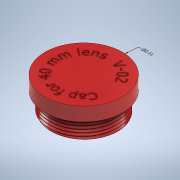
# Autodesk Inventor part: CapForSvBonyPlosse-40mm-V02
Saved by Autodesk Inventor 2021.1 (Build 251245010, 245A)
## iProperties
Created: 2020-10-08
Part Number: CapForSvBonyPlosse-40mm-V02
Material: PC/ABS Plastic
Document SubType Name: Modeling
Designer: robst
Density: 0.357273 g/cm^3
Appearance: Red
Author: robst
Autodesk Inventor part; units mm, degrees
ref_plane "YZ Plane" through (0, 0, 0) normal (1, 0, 0) x (0, 1, 0)
ref_plane "XZ Plane" through (0, 0, 0) normal (0, 1, 0) x (-1, 0, 0)
ref_plane "XY Plane" through (0, 0, 0) normal (0, 0, 1) x (1, 0, 0)
sketch "Sketch7" plane through (0, 0, 0) normal (0, 0, 1) x (1, 0, 0)
  line L0 (0, 0) -> (23.5712, 0)
  line L1 (23.5712, 0) -> (23.5712, 12.7)
  line L2 (23.5712, 12.7) -> (26.7462, 12.7)
  line L3 (26.7462, 12.7) -> (26.7462, 22.225)
  line L4 (26.7462, 22.225) -> (0, 22.225)
  line L5 (23.5712, 0) -> (20.3962, 0)
  line L6 (20.3962, 0) -> (20.3962, 19.05)
  line L7 (20.3962, 19.05) -> (0, 19.05)
  line L8 (0, 22.225) -> (0, 19.05)
  line L9 (0, -4.445) -> (0, 26.67) projected
  dimension "d71" = 9.525
  dimension "d72" = 12.7
  dimension "d73" = 23.5712
  dimension "d77" = 3.175
  dimension "d78" = 3.175
  dimension "d117" = 20.3962
  constraints: 18 end point, 5 perpendicular, 2 vertical, 1 horizontal, 1 point on line
  measures "d71" distance between parallel lines of L4 L2
  measures "d72" distance from line of L2 L0.start
  measures "d73" distance of L0.start L0.end
  measures "d77" distance of L2.end L1.end
  measures "d78" distance between parallel lines of L1 L6
  measures "d117" distance between parallel lines of L6 L9
revolve "Revolution3" add sketch "Sketch7" angle 360 about axis through (0, -10, 0) along (0, 1, 0) contours L6 L7 L8 L4 L3 L2 L1 L0
sketch "Sketch10" plane through (0, 0, 0) normal (0, 0, 1) x (1, 0, 0)
  line L0 (23.5712, 12.7) -> (23.5712, 0) projected
  line L1 (23.5712, -2.1167) -> (23.5712, -4.0025)
  line L2 (23.5712, -4.0025) -> (22.3266, -3.284)
  line L3 (22.3266, -2.8352) -> (23.5712, -2.1167)
  line L4 (-23.5712, 0) -> (23.5712, 0) projected
  arc A0 (22.3266, -2.8352) -> (22.3266, -3.284) centre (22.4561, -3.0596) ccw
  line L5 (0, -7.3431) -> (0, 16.0405) projected
  point P0 (0, 0)
  dimension "d100" = 60
  dimension "d101" = 2.1167
  dimension "d102" = 0.2591
  dimension "d103" = 22.1971
  constraints: 6 end point, 2 point on circle, 2 tangent, 1 centre point, 1 collinear, 1 equal length, 1 vertical
  measures "d100" angle of L3 L2
  measures "d101" distance from line of L1.start L4
  measures "d102" radius of A0
  measures "d103" distance edge to line of A0 L5
coil "Coil6" sketch "Sketch10" operation cut axis through (0, -10, 0) along (0, 1, 0) pitch 2.1167 turns 8 hand right
sketch "Sketch11" plane through (0, 22.225, 0) normal (0, 1, 0) x (1, 0, 0)
  circle A0 centre (0, 0) radius 19.05 construction
  spline S0 degree 2 poles (13.5686, -8.6606) (13.8543, -8.1839) (14.6595, -7.5704) (15.1574, -7.4694) knots 0 0 0 1 2 2 2
  spline S1 degree 2 poles (15.1574, -7.4694) (15.6514, -7.3659) (16.7976, -7.6157) (17.4173, -7.9871) knots 0 0 0 1 2 2 2
  spline S2 degree 2 poles (17.4173, -7.9871) (18.033, -8.3562) (18.7585, -9.2177) (18.9175, -9.718) knots 0 0 0 1 2 2 2
  spline S3 degree 2 poles (18.9175, -9.718) (19.071, -10.2096) (18.9356, -11.2192) (18.6379, -11.7157) knots 0 0 0 1 2 2 2
  spline S4 degree 2 poles (18.6379, -11.7157) (18.4903, -11.962) (18.1592, -12.3521) (17.9941, -12.5015) knots 0 0 0 1 2 2 2
  spline S5 degree 2 poles (17.9941, -12.5015) (17.8472, -12.6294) (17.5026, -12.871) (17.3175, -12.9815) knots 0 0 0 1 2 2 2
  line L0 (17.3175, -12.9815) -> (16.5311, -12.51)
  line L1 (16.5311, -12.51) -> (16.562, -12.4583)
  spline S6 degree 2 poles (16.562, -12.4583) (16.6938, -12.4186) (17.0782, -12.2818) (17.3021, -12.1515) knots 0 0 0 1 2 2 2
  spline S7 degree 2 poles (17.3021, -12.1515) (17.5173, -12.0267) (17.9127, -11.6644) (18.0842, -11.3784) knots 0 0 0 1 2 2 2
  spline S8 degree 2 poles (18.0842, -11.3784) (18.2723, -11.0646) (18.3499, -10.3497) (18.2298, -9.9915) knots 0 0 0 1 2 2 2
  spline S9 degree 2 poles (18.2298, -9.9915) (18.1034, -9.635) (17.4828, -8.9498) (17.0101, -8.6664) knots 0 0 0 1 2 2 2
  spline S10 degree 2 poles (17.0101, -8.6664) (16.5056, -8.364) (15.6335, -8.1705) (15.257, -8.231) knots 0 0 0 1 2 2 2
  spline S11 degree 2 poles (15.257, -8.231) (14.8909, -8.2923) (14.3136, -8.6968) (14.1279, -9.0066) knots 0 0 0 1 2 2 2
  spline S12 degree 2 poles (14.1279, -9.0066) (13.9588, -9.2887) (13.8097, -9.8526) (13.8011, -10.1012) knots 0 0 0 1 2 2 2
  spline S13 degree 2 poles (13.8011, -10.1012) (13.7972, -10.3419) (13.8521, -10.7366) (13.8824, -10.8574) knots 0 0 0 1 2 2 2
  line L2 (13.8824, -10.8574) -> (13.8538, -10.905)
  line L3 (13.8538, -10.905) -> (13.0752, -10.4383)
  spline S14 degree 2 poles (13.0752, -10.4383) (13.0974, -10.2302) (13.1298, -9.8608) (13.1877, -9.6202) knots 0 0 0 1 2 2 2
  spline S15 degree 2 poles (13.1877, -9.6202) (13.2448, -9.3628) (13.3924, -8.9545) (13.5686, -8.6606) knots 0 0 0 1 2 2 2
  spline S16 degree 2 poles (10.8434, -12.6588) (10.8626, -12.5511) (10.9182, -12.1791) (10.9711, -12.0331) knots 0 0 0 1 2 2 2
  spline S17 degree 2 poles (10.9711, -12.0331) (11.0387, -11.8285) (11.224, -11.5057) (11.4592, -11.2825) knots 0 0 0 1 2 2 2
  spline S18 degree 2 poles (11.4592, -11.2825) (11.6506, -11.1008) (12.1337, -10.9169) (12.3891, -10.9235) knots 0 0 0 1 2 2 2
  spline S19 degree 2 poles (12.3891, -10.9235) (12.6345, -10.9332) (13.1427, -11.1659) (13.3404, -11.3742) knots 0 0 0 1 2 2 2
  spline S20 degree 2 poles (13.3404, -11.3742) (13.6465, -11.6967) (13.808, -12.4118) (13.6368, -12.8233) knots 0 0 0 1 2 2 2
  spline S21 degree 2 poles (13.6368, -12.8233) (13.4895, -13.193) (12.8635, -13.9596) (12.4726, -14.3753) knots 0 0 0 1 2 2 2
  line L4 (12.4726, -14.3753) -> (12.5683, -14.476)
  spline S22 degree 2 poles (12.5683, -14.476) (12.7405, -14.6574) (13.0649, -14.7773) (13.2263, -14.7454) knots 0 0 0 1 2 2 2
  spline S23 degree 2 poles (13.2263, -14.7454) (13.3876, -14.7136) (13.7148, -14.4797) (13.8693, -14.3331) knots 0 0 0 1 2 2 2
  spline S24 degree 2 poles (13.8693, -14.3331) (14.0507, -14.1609) (14.4391, -13.5879) (14.5854, -13.251) knots 0 0 0 1 2 2 2
  line L5 (14.5854, -13.251) -> (14.6157, -13.2223)
  line L6 (14.6157, -13.2223) -> (15.1226, -13.7564)
  spline S25 degree 2 poles (15.1226, -13.7564) (15.0164, -13.9338) (14.5713, -14.5479) (14.3059, -14.7998) knots 0 0 0 1 2 2 2
  spline S26 degree 2 poles (14.3059, -14.7998) (13.9834, -15.1059) (13.4477, -15.4228) (13.1487, -15.4576) knots 0 0 0 1 2 2 2
  spline S27 degree 2 poles (13.1487, -15.4576) (12.8563, -15.4925) (12.3025, -15.2455) (12.0251, -14.9532) knots 0 0 0 1 2 2 2
  line L7 (12.0251, -14.9532) -> (10.0069, -12.8269)
  line L8 (10.0069, -12.8269) -> (10.531, -12.3296)
  line L9 (10.531, -12.3296) -> (10.8434, -12.6588)
  line L10 (11.2579, -13.0954) -> (12.0773, -13.9587)
  spline S28 degree 2 poles (12.0773, -13.9587) (12.2495, -13.7634) (12.7629, -13.1675) (12.89, -12.9447) knots 0 0 0 1 2 2 2
  spline S29 degree 2 poles (12.89, -12.9447) (13.0376, -12.6832) (13.0579, -12.1596) (12.8347, -11.9245) knots 0 0 0 1 2 2 2
  spline S30 degree 2 poles (12.8347, -11.9245) (12.5796, -11.6557) (12.019, -11.6706) (11.7302, -11.9448) knots 0 0 0 1 2 2 2
  spline S31 degree 2 poles (11.7302, -11.9448) (11.4849, -12.1775) (11.2827, -12.7718) (11.2579, -13.0954) knots 0 0 0 1 2 2 2
  spline S32 degree 2 poles (7.1265, -17.1316) (6.6121, -16.1883) (6.9032, -14.5842) (7.5904, -14.2095) knots 0 0 0 1 2 2 2
  spline S33 degree 2 poles (7.5904, -14.2095) (7.8709, -14.0565) (8.3729, -13.9516) (8.6697, -13.9638) knots 0 0 0 1 2 2 2
  line L11 (8.6697, -13.9638) -> (7.8094, -12.3862)
  line L12 (7.8094, -12.3862) -> (8.4437, -12.0403)
  line L13 (8.4437, -12.0403) -> (11.2529, -17.192)
  line L14 (11.2529, -17.192) -> (10.6186, -17.5379)
  line L15 (10.6186, -17.5379) -> (10.4036, -17.1435)
  spline S34 degree 2 poles (10.4036, -17.1435) (10.2853, -17.4876) (9.8631, -18.087) (9.5256, -18.2711) knots 0 0 0 1 2 2 2
  spline S35 degree 2 poles (9.5256, -18.2711) (8.8791, -18.6236) (7.5966, -17.9936) (7.1265, -17.1316) knots 0 0 0 1 2 2 2
  spline S36 degree 2 poles (7.7413, -16.7015) (8.0938, -17.348) (8.8925, -17.8356) (9.352, -17.585) knots 0 0 0 1 2 2 2
  spline S37 degree 2 poles (9.352, -17.585) (9.6203, -17.4387) (9.9937, -16.9239) (10.1153, -16.6149) knots 0 0 0 1 2 2 2
  line L16 (10.1153, -16.6149) -> (8.949, -14.4761)
  spline S38 degree 2 poles (8.949, -14.4761) (8.6367, -14.4935) (8.2342, -14.5969) (8.0065, -14.7211) knots 0 0 0 1 2 2 2
  spline S39 degree 2 poles (8.0065, -14.7211) (7.5145, -14.9894) (7.3643, -16.0102) (7.7413, -16.7015) knots 0 0 0 1 2 2 2
  line L17 (1.4019, -21.4704) -> (1.4386, -21.4655)
  spline S40 degree 2 poles (1.4386, -21.4655) (1.5399, -21.4894) (1.9065, -21.506) (2.0488, -21.487) knots 0 0 0 1 2 2 2
  spline S41 degree 2 poles (2.0488, -21.487) (2.4987, -21.4271) (2.8306, -20.9717) (2.7596, -20.4392) knots 0 0 0 1 2 2 2
  line L18 (2.7596, -20.4392) -> (2.7407, -20.2969)
  line L19 (2.7407, -20.2969) -> (1.5563, -20.4546)
  line L20 (1.5563, -20.4546) -> (1.4774, -19.8624)
  line L21 (1.4774, -19.8624) -> (2.6388, -19.7078)
  line L22 (2.6388, -19.7078) -> (2.1515, -16.0489)
  line L23 (2.1515, -16.0489) -> (2.8677, -15.9535)
  line L24 (2.8677, -15.9535) -> (3.355, -19.6124)
  line L25 (3.355, -19.6124) -> (3.837, -19.5482)
  line L26 (3.837, -19.5482) -> (3.9159, -20.1404)
  line L27 (3.9159, -20.1404) -> (3.4339, -20.2046)
  line L28 (3.4339, -20.2046) -> (3.4528, -20.3469)
  spline S42 degree 2 poles (3.4528, -20.3469) (3.5543, -21.109) (2.9216, -22.0062) (2.233, -22.0979) knots 0 0 0 1 2 2 2
  spline S43 degree 2 poles (2.233, -22.0979) (2.0356, -22.1242) (1.6491, -22.1336) (1.4893, -22.1269) knots 0 0 0 1 2 2 2
  line L29 (1.4893, -22.1269) -> (1.4019, -21.4704)
  spline S44 degree 2 poles (-3.3876, -18.1226) (-3.3002, -17.0424) (-2.1663, -15.9493) (-1.2985, -16.0195) knots 0 0 0 1 2 2 2
  spline S45 degree 2 poles (-1.2985, -16.0195) (-0.4075, -16.0916) (0.5144, -17.3882) (0.43, -18.4315) knots 0 0 0 1 2 2 2
  spline S46 degree 2 poles (0.43, -18.4315) (0.3434, -19.5025) (-0.8051, -20.6037) (-1.6637, -20.5342) knots 0 0 0 1 2 2 2
  spline S47 degree 2 poles (-1.6637, -20.5342) (-2.5316, -20.464) (-3.4746, -19.1982) (-3.3876, -18.1226) knots 0 0 0 1 2 2 2
  spline S48 degree 2 poles (-2.6444, -18.1827) (-2.7116, -19.0137) (-2.1722, -19.8704) (-1.6137, -19.9156) knots 0 0 0 1 2 2 2
  spline S49 degree 2 poles (-1.6137, -19.9156) (-1.0551, -19.9608) (-0.3804, -19.2023) (-0.3132, -18.3714) knots 0 0 0 1 2 2 2
  spline S50 degree 2 poles (-0.3132, -18.3714) (-0.2478, -17.5635) (-0.7899, -16.6833) (-1.3485, -16.6381) knots 0 0 0 1 2 2 2
  spline S51 degree 2 poles (-1.3485, -16.6381) (-1.9025, -16.5933) (-2.5779, -17.3611) (-2.6444, -18.1827) knots 0 0 0 1 2 2 2
  line L30 (-7.1238, -18.4268) -> (-7.0884, -18.4377)
  spline S52 degree 2 poles (-7.0884, -18.4377) (-7.0156, -18.4844) (-6.8457, -18.5465) (-6.7262, -18.5833) knots 0 0 0 1 2 2 2
  spline S53 degree 2 poles (-6.7262, -18.5833) (-6.4474, -18.6692) (-5.8235, -18.595) (-5.502, -18.4324) knots 0 0 0 1 2 2 2
  line L31 (-5.502, -18.4324) -> (-4.6058, -15.5246)
  line L32 (-4.6058, -15.5246) -> (-3.9154, -15.7374)
  line L33 (-3.9154, -15.7374) -> (-5.1786, -19.8357)
  line L34 (-5.1786, -19.8357) -> (-5.869, -19.6229)
  line L35 (-5.869, -19.6229) -> (-5.6807, -19.0121)
  spline S54 degree 2 poles (-5.6807, -19.0121) (-6.1606, -19.2325) (-6.8073, -19.3337) (-7.0728, -19.2519) knots 0 0 0 1 2 2 2
  spline S55 degree 2 poles (-7.0728, -19.2519) (-7.179, -19.2191) (-7.2825, -19.1775) (-7.3448, -19.1438) knots 0 0 0 1 2 2 2
  line L36 (-7.3448, -19.1438) -> (-7.1238, -18.4268)
  line L37 (-12.7931, -13.0301) -> (-12.2592, -13.4525)
  line L38 (-12.2592, -13.4525) -> (-11.0409, -11.9124)
  line L39 (-11.0409, -11.9124) -> (-10.4634, -12.3692)
  line L40 (-10.4634, -12.3692) -> (-11.6816, -13.9093)
  line L41 (-11.6816, -13.9093) -> (-9.702, -15.4752)
  line L42 (-9.702, -15.4752) -> (-10.202, -16.1072)
  line L43 (-10.202, -16.1072) -> (-14.0344, -16.8314)
  line L44 (-14.0344, -16.8314) -> (-14.5865, -16.3946)
  line L45 (-14.5865, -16.3946) -> (-12.6413, -13.9356)
  line L46 (-12.6413, -13.9356) -> (-13.1753, -13.5132)
  line L47 (-13.1753, -13.5132) -> (-12.7931, -13.0301)
  line L48 (-12.0638, -14.3924) -> (-13.4487, -16.1432)
  line L49 (-13.4487, -16.1432) -> (-10.5564, -15.5848)
  line L50 (-10.5564, -15.5848) -> (-12.0638, -14.3924)
  spline S56 degree 2 poles (-16.3898, -9.8804) (-15.1549, -8.9643) (-13.4656, -8.8241) (-12.911, -9.5717) knots 0 0 0 1 2 2 2
  spline S57 degree 2 poles (-12.911, -9.5717) (-12.3481, -10.3305) (-13.0002, -11.9156) (-14.2091, -12.8124) knots 0 0 0 1 2 2 2
  spline S58 degree 2 poles (-14.2091, -12.8124) (-15.4514, -13.734) (-17.1333, -13.8687) (-17.6907, -13.1173) knots 0 0 0 1 2 2 2
  spline S59 degree 2 poles (-17.6907, -13.1173) (-18.2508, -12.3623) (-17.5876, -10.7689) (-16.3898, -9.8804) knots 0 0 0 1 2 2 2
  spline S60 degree 2 poles (-14.4063, -9.6315) (-14.6994, -9.7105) (-15.4539, -10.1549) (-15.9263, -10.5053) knots 0 0 0 1 2 2 2
  spline S61 degree 2 poles (-15.9263, -10.5053) (-16.3987, -10.8557) (-17.0391, -11.4461) (-17.2044, -11.7129) knots 0 0 0 1 2 2 2
  spline S62 degree 2 poles (-17.2044, -11.7129) (-17.3698, -11.9797) (-17.3715, -12.4827) (-17.1811, -12.7393) knots 0 0 0 1 2 2 2
  spline S63 degree 2 poles (-17.1811, -12.7393) (-16.9907, -12.996) (-16.5034, -13.1477) (-16.1899, -13.065) knots 0 0 0 1 2 2 2
  spline S64 degree 2 poles (-16.1899, -13.065) (-15.8865, -12.9842) (-15.1227, -12.5214) (-14.6726, -12.1875) knots 0 0 0 1 2 2 2
  spline S65 degree 2 poles (-14.6726, -12.1875) (-14.1891, -11.8288) (-13.586, -11.2892) (-13.4048, -11.0048) knots 0 0 0 1 2 2 2
  spline S66 degree 2 poles (-13.4048, -11.0048) (-13.233, -10.739) (-13.2219, -10.2176) (-13.4206, -9.9497) knots 0 0 0 1 2 2 2
  spline S67 degree 2 poles (-13.4206, -9.9497) (-13.6082, -9.6968) (-14.0956, -9.5451) (-14.4063, -9.6315) knots 0 0 0 1 2 2 2
  line L51 (-16.3208, -0.4262) -> (-18.7737, -0.8076)
  spline S68 degree 2 poles (-18.7737, -0.8076) (-19.0666, -0.8531) (-19.5583, -0.9764) (-19.6842, -1.071) knots 0 0 0 1 2 2 2
  spline S69 degree 2 poles (-19.6842, -1.071) (-19.8238, -1.1677) (-19.9269, -1.4696) (-19.8891, -1.7121) knots 0 0 0 1 2 2 2
  spline S70 degree 2 poles (-19.8891, -1.7121) (-19.855, -1.9318) (-19.5067, -2.3932) (-19.2092, -2.6188) knots 0 0 0 1 2 2 2
  spline S71 degree 2 poles (-19.2092, -2.6188) (-19.1458, -2.6043) (-18.9688, -2.5674) (-18.8498, -2.5489) knots 0 0 0 1 2 2 2
  line L52 (-18.8498, -2.5489) -> (-16.0582, -2.1148)
  line L53 (-16.0582, -2.1148) -> (-15.9472, -2.8287)
  line L54 (-15.9472, -2.8287) -> (-18.4001, -3.2101)
  spline S72 degree 2 poles (-18.4001, -3.2101) (-18.693, -3.2556) (-19.1847, -3.379) (-19.3106, -3.4735) knots 0 0 0 1 2 2 2
  spline S73 degree 2 poles (-19.3106, -3.4735) (-19.4503, -3.5702) (-19.5533, -3.8722) (-19.5156, -4.1147) knots 0 0 0 1 2 2 2
  spline S74 degree 2 poles (-19.5156, -4.1147) (-19.48, -4.3435) (-19.1127, -4.8067) (-18.8515, -5.0098) knots 0 0 0 1 2 2 2
  line L55 (-18.8515, -5.0098) -> (-15.6847, -4.5174)
  line L56 (-15.6847, -4.5174) -> (-15.5737, -5.2313)
  line L57 (-15.5737, -5.2313) -> (-19.8113, -5.8902)
  line L58 (-19.8113, -5.8902) -> (-19.9223, -5.1763)
  line L59 (-19.9223, -5.1763) -> (-19.4555, -5.1037)
  spline S75 degree 2 poles (-19.4555, -5.1037) (-19.7781, -4.8679) (-20.1701, -4.3665) (-20.2213, -4.037) knots 0 0 0 1 2 2 2
  spline S76 degree 2 poles (-20.2213, -4.037) (-20.2797, -3.6617) (-20.0268, -3.0271) (-19.6613, -2.8156) knots 0 0 0 1 2 2 2
  spline S77 degree 2 poles (-19.6613, -2.8156) (-20.0734, -2.5469) (-20.5394, -1.9914) (-20.5949, -1.6344) knots 0 0 0 1 2 2 2
  spline S78 degree 2 poles (-20.5949, -1.6344) (-20.6376, -1.3598) (-20.538, -0.885) (-20.3714, -0.6904) knots 0 0 0 1 2 2 2
  spline S79 degree 2 poles (-20.3714, -0.6904) (-20.2055, -0.4912) (-19.6581, -0.2139) (-19.2233, -0.1463) knots 0 0 0 1 2 2 2
  line L60 (-19.2233, -0.1463) -> (-16.4318, 0.2877)
  line L61 (-16.4318, 0.2877) -> (-16.3208, -0.4262)
  line L62 (-15.1861, 5.9945) -> (-17.5926, 6.6033)
  spline S80 degree 2 poles (-17.5926, 6.6033) (-17.8799, 6.6761) (-18.3807, 6.755) (-18.5336, 6.7172) knots 0 0 0 1 2 2 2
  spline S81 degree 2 poles (-18.5336, 6.7172) (-18.6999, 6.6829) (-18.9129, 6.4453) (-18.9731, 6.2074) knots 0 0 0 1 2 2 2
  spline S82 degree 2 poles (-18.9731, 6.2074) (-19.0276, 5.9919) (-18.8877, 5.431) (-18.7021, 5.107) knots 0 0 0 1 2 2 2
  spline S83 degree 2 poles (-18.7021, 5.107) (-18.6381, 5.0955) (-18.4608, 5.0602) (-18.344, 5.0307) knots 0 0 0 1 2 2 2
  line L63 (-18.344, 5.0307) -> (-15.6052, 4.3377)
  line L64 (-15.6052, 4.3377) -> (-15.7825, 3.6373)
  line L65 (-15.7825, 3.6373) -> (-18.189, 4.2462)
  spline S84 degree 2 poles (-18.189, 4.2462) (-18.4763, 4.3189) (-18.9771, 4.3978) (-19.13, 4.3601) knots 0 0 0 1 2 2 2
  spline S85 degree 2 poles (-19.13, 4.3601) (-19.2963, 4.3257) (-19.5093, 4.0882) (-19.5695, 3.8502) knots 0 0 0 1 2 2 2
  spline S86 degree 2 poles (-19.5695, 3.8502) (-19.6263, 3.6258) (-19.4695, 3.0558) (-19.3086, 2.7667) knots 0 0 0 1 2 2 2
  line L66 (-19.3086, 2.7667) -> (-16.2016, 1.9806)
  line L67 (-16.2016, 1.9806) -> (-16.3789, 1.2802)
  line L68 (-16.3789, 1.2802) -> (-20.5364, 2.3321)
  line L69 (-20.5364, 2.3321) -> (-20.3592, 3.0325)
  line L70 (-20.3592, 3.0325) -> (-19.9012, 2.9166)
  spline S87 degree 2 poles (-19.9012, 2.9166) (-20.1058, 3.2598) (-20.2703, 3.8747) (-20.1885, 4.198) knots 0 0 0 1 2 2 2
  spline S88 degree 2 poles (-20.1885, 4.198) (-20.0954, 4.5661) (-19.6144, 5.0511) (-19.1952, 5.1027) knots 0 0 0 1 2 2 2
  spline S89 degree 2 poles (-19.1952, 5.1027) (-19.4693, 5.5113) (-19.6807, 6.2049) (-19.5921, 6.5551) knots 0 0 0 1 2 2 2
  spline S90 degree 2 poles (-19.5921, 6.5551) (-19.524, 6.8245) (-19.2465, 7.2225) (-19.0171, 7.3364) knots 0 0 0 1 2 2 2
  spline S91 degree 2 poles (-19.0171, 7.3364) (-18.7864, 7.4548) (-18.1742, 7.4957) (-17.7476, 7.3878) knots 0 0 0 1 2 2 2
  line L71 (-17.7476, 7.3878) -> (-15.0089, 6.6949)
  line L72 (-15.0089, 6.6949) -> (-15.1861, 5.9945)
  line L73 (-12.6155, 10.1576) -> (-13.056, 9.5848)
  line L74 (-13.056, 9.5848) -> (-17.7881, 13.2241)
  line L75 (-17.7881, 13.2241) -> (-17.3477, 13.7968)
  line L76 (-17.3477, 13.7968) -> (-12.6155, 10.1576)
  spline S92 degree 2 poles (-10.5308, 12.1762) (-11.2951, 11.4884) (-12.9065, 11.5897) (-13.619, 12.3815) knots 0 0 0 1 2 2 2
  spline S93 degree 2 poles (-13.619, 12.3815) (-14.3192, 13.1595) (-14.3335, 14.8163) (-13.676, 15.408) knots 0 0 0 1 2 2 2
  spline S94 degree 2 poles (-13.676, 15.408) (-13.38, 15.6745) (-12.7672, 15.9144) (-12.4343, 15.8837) knots 0 0 0 1 2 2 2
  spline S95 degree 2 poles (-12.4343, 15.8837) (-12.098, 15.8562) (-11.4416, 15.4936) (-11.0977, 15.1115) knots 0 0 0 1 2 2 2
  line L77 (-11.0977, 15.1115) -> (-10.8343, 14.8189)
  line L78 (-10.8343, 14.8189) -> (-13.041, 12.8331)
  spline S96 degree 2 poles (-13.041, 12.8331) (-12.5422, 12.2788) (-11.4548, 12.192) (-10.9591, 12.6382) knots 0 0 0 1 2 2 2
  spline S97 degree 2 poles (-10.9591, 12.6382) (-10.7835, 12.7962) (-10.5139, 13.182) (-10.432, 13.3679) knots 0 0 0 1 2 2 2
  spline S98 degree 2 poles (-10.432, 13.3679) (-10.3494, 13.5669) (-10.2581, 13.8671) (-10.2423, 13.981) knots 0 0 0 1 2 2 2
  line L79 (-10.2423, 13.981) -> (-10.2113, 14.0089)
  line L80 (-10.2113, 14.0089) -> (-9.6846, 13.4237)
  spline S99 degree 2 poles (-9.6846, 13.4237) (-9.7435, 13.3021) (-9.9267, 12.9379) (-10.0089, 12.8078) knots 0 0 0 1 2 2 2
  spline S100 degree 2 poles (-10.0089, 12.8078) (-10.1236, 12.6237) (-10.3381, 12.3497) (-10.5308, 12.1762) knots 0 0 0 1 2 2 2
  spline S101 degree 2 poles (-11.7263, 14.7577) (-11.9283, 14.9684) (-12.3029, 15.2045) (-12.485, 15.2338) knots 0 0 0 1 2 2 2
  spline S102 degree 2 poles (-12.485, 15.2338) (-12.6863, 15.2706) (-13.0936, 15.1347) (-13.3105, 14.9395) knots 0 0 0 1 2 2 2
  spline S103 degree 2 poles (-13.3105, 14.9395) (-13.5239, 14.7474) (-13.7088, 14.3505) (-13.7212, 14.1151) knots 0 0 0 1 2 2 2
  spline S104 degree 2 poles (-13.7212, 14.1151) (-13.727, 13.8793) (-13.5752, 13.4613) (-13.4097, 13.2427) knots 0 0 0 1 2 2 2
  line L81 (-13.4097, 13.2427) -> (-11.7263, 14.7577)
  line L82 (-5.8376, 15.199) -> (-6.4813, 14.8709)
  line L83 (-6.4813, 14.8709) -> (-7.5915, 17.0497)
  spline S105 degree 2 poles (-7.5915, 17.0497) (-7.7261, 17.3138) (-8.0069, 17.7424) (-8.1506, 17.8408) knots 0 0 0 1 2 2 2
  spline S106 degree 2 poles (-8.1506, 17.8408) (-8.3026, 17.9452) (-8.6547, 17.9426) (-8.894, 17.8206) knots 0 0 0 1 2 2 2
  spline S107 degree 2 poles (-8.894, 17.8206) (-9.1333, 17.6986) (-9.5105, 17.1842) (-9.6488, 16.8538) knots 0 0 0 1 2 2 2
  line L84 (-9.6488, 16.8538) -> (-8.1937, 13.9983)
  line L85 (-8.1937, 13.9983) -> (-8.8374, 13.6703)
  line L86 (-8.8374, 13.6703) -> (-10.7846, 17.4913)
  line L87 (-10.7846, 17.4913) -> (-10.1409, 17.8194)
  line L88 (-10.1409, 17.8194) -> (-9.9243, 17.3943)
  spline S108 degree 2 poles (-9.9243, 17.3943) (-9.7679, 17.8015) (-9.3496, 18.3577) (-9.036, 18.5175) knots 0 0 0 1 2 2 2
  spline S109 degree 2 poles (-9.036, 18.5175) (-8.4748, 18.8035) (-7.4609, 18.3846) (-7.1013, 17.6789) knots 0 0 0 1 2 2 2
  line L89 (-7.1013, 17.6789) -> (-5.8376, 15.199)
  spline S110 degree 2 poles (-3.7223, 15.6543) (-4.1417, 15.5566) (-4.9205, 15.6128) (-5.189, 15.6834) knots 0 0 0 1 2 2 2
  line L90 (-5.189, 15.6834) -> (-5.3729, 16.4727)
  line L91 (-5.3729, 16.4727) -> (-5.3368, 16.4811)
  spline S111 degree 2 poles (-5.3368, 16.4811) (-5.2298, 16.43) (-4.9463, 16.3154) (-4.7213, 16.2679) knots 0 0 0 1 2 2 2
  spline S112 degree 2 poles (-4.7213, 16.2679) (-4.5254, 16.2232) (-4.063, 16.1979) (-3.8329, 16.2515) knots 0 0 0 1 2 2 2
  spline S113 degree 2 poles (-3.8329, 16.2515) (-3.666, 16.2904) (-3.3005, 16.4564) (-3.225, 16.5406) knots 0 0 0 1 2 2 2
  spline S114 degree 2 poles (-3.225, 16.5406) (-3.1142, 16.6568) (-3.0421, 16.878) (-3.0884, 17.0765) knots 0 0 0 1 2 2 2
  spline S115 degree 2 poles (-3.0884, 17.0765) (-3.1462, 17.3246) (-3.4768, 17.5186) (-3.844, 17.5233) knots 0 0 0 1 2 2 2
  spline S116 degree 2 poles (-3.844, 17.5233) (-3.9867, 17.5234) (-4.4407, 17.5127) (-4.6372, 17.5192) knots 0 0 0 1 2 2 2
  spline S117 degree 2 poles (-4.6372, 17.5192) (-5.1479, 17.5476) (-5.7155, 18.024) (-5.8111, 18.4344) knots 0 0 0 1 2 2 2
  spline S118 degree 2 poles (-5.8111, 18.4344) (-5.9436, 19.0027) (-5.2562, 19.9096) (-4.5525, 20.0736) knots 0 0 0 1 2 2 2
  spline S119 degree 2 poles (-4.5525, 20.0736) (-4.2052, 20.1545) (-3.4617, 20.1471) (-3.1921, 20.072) knots 0 0 0 1 2 2 2
  line L92 (-3.1921, 20.072) -> (-3.0166, 19.3188)
  line L93 (-3.0166, 19.3188) -> (-3.0527, 19.3104)
  spline S120 degree 2 poles (-3.0527, 19.3104) (-3.3737, 19.4638) (-4.0901, 19.5584) (-4.4284, 19.4795) knots 0 0 0 1 2 2 2
  spline S121 degree 2 poles (-4.4284, 19.4795) (-4.7757, 19.3986) (-5.1854, 18.994) (-5.1171, 18.7008) knots 0 0 0 1 2 2 2
  spline S122 degree 2 poles (-5.1171, 18.7008) (-5.0551, 18.4347) (-4.711, 18.2438) (-4.3763, 18.2362) knots 0 0 0 1 2 2 2
  spline S123 degree 2 poles (-4.3763, 18.2362) (-4.2135, 18.2314) (-3.8067, 18.2406) (-3.5832, 18.2404) knots 0 0 0 1 2 2 2
  spline S124 degree 2 poles (-3.5832, 18.2404) (-3.0958, 18.2303) (-2.5016, 17.8029) (-2.3933, 17.3384) knots 0 0 0 1 2 2 2
  spline S125 degree 2 poles (-2.3933, 17.3384) (-2.3302, 17.0677) (-2.4308, 16.5402) (-2.5973, 16.316) knots 0 0 0 1 2 2 2
  spline S126 degree 2 poles (-2.5973, 16.316) (-2.7752, 16.0795) (-3.2938, 15.7542) (-3.7223, 15.6543) knots 0 0 0 1 2 2 2
  line L94 (9.2637, 19.9906) -> (5.5627, 15.2117)
  line L95 (5.5627, 15.2117) -> (4.7865, 15.4752)
  line L96 (4.7865, 15.4752) -> (4.7598, 21.5196)
  line L97 (4.7598, 21.5196) -> (5.5317, 21.2576)
  line L98 (5.5317, 21.2576) -> (5.5055, 16.2533)
  line L99 (5.5055, 16.2533) -> (8.5313, 20.2392)
  line L100 (8.5313, 20.2392) -> (9.2637, 19.9906)
  line L101 (10.6778, 14.9578) -> (8.8465, 16.1084)
  line L102 (8.8465, 16.1084) -> (9.2161, 16.6967)
  line L103 (9.2161, 16.6967) -> (11.0474, 15.546)
  line L104 (11.0474, 15.546) -> (10.6778, 14.9578)
  spline S127 degree 2 poles (14.704, 12.2491) (13.6221, 11.1566) (11.9735, 10.7621) (11.3121, 11.4171) knots 0 0 0 1 2 2 2
  spline S128 degree 2 poles (11.3121, 11.4171) (10.6407, 12.0818) (11.0452, 13.7474) (12.1043, 14.817) knots 0 0 0 1 2 2 2
  spline S129 degree 2 poles (12.1043, 14.817) (13.1927, 15.9161) (14.8347, 16.3041) (15.4995, 15.6458) knots 0 0 0 1 2 2 2
  spline S130 degree 2 poles (15.4995, 15.6458) (16.1675, 14.9843) (15.7533, 13.3088) (14.704, 12.2491) knots 0 0 0 1 2 2 2
  spline S131 degree 2 poles (12.7811, 11.7026) (13.0588, 11.8252) (13.7373, 12.3787) (14.1511, 12.7966) knots 0 0 0 1 2 2 2
  spline S132 degree 2 poles (14.1511, 12.7966) (14.565, 13.2145) (15.1085, 13.8951) (15.2316, 14.1839) knots 0 0 0 1 2 2 2
  spline S133 degree 2 poles (15.2316, 14.1839) (15.3546, 14.4727) (15.2801, 14.9701) (15.053, 15.1949) knots 0 0 0 1 2 2 2
  spline S134 degree 2 poles (15.053, 15.1949) (14.826, 15.4198) (14.3213, 15.4959) (14.0239, 15.3667) knots 0 0 0 1 2 2 2
  spline S135 degree 2 poles (14.0239, 15.3667) (13.7363, 15.2409) (13.0514, 14.6677) (12.6571, 14.2695) knots 0 0 0 1 2 2 2
  spline S136 degree 2 poles (12.6571, 14.2695) (12.2335, 13.8417) (11.7191, 13.217) (11.5831, 12.9084) knots 0 0 0 1 2 2 2
  spline S137 degree 2 poles (11.5831, 12.9084) (11.4535, 12.6196) (11.5216, 12.1025) (11.7585, 11.8679) knots 0 0 0 1 2 2 2
  spline S138 degree 2 poles (11.7585, 11.8679) (11.9823, 11.6463) (12.487, 11.5702) (12.7811, 11.7026) knots 0 0 0 1 2 2 2
  line L105 (14.8993, 6.5906) -> (13.1268, 9.6368)
  line L106 (13.1268, 9.6368) -> (13.8273, 10.0445)
  spline S139 degree 2 poles (13.8273, 10.0445) (14.3265, 9.8956) (15.239, 9.6442) (15.7103, 9.5434) knots 0 0 0 1 2 2 2
  spline S140 degree 2 poles (15.7103, 9.5434) (16.6592, 9.34) (17.6436, 9.3609) (18.0399, 9.5915) knots 0 0 0 1 2 2 2
  spline S141 degree 2 poles (18.0399, 9.5915) (18.2481, 9.7126) (18.4857, 10.0224) (18.5183, 10.1967) knots 0 0 0 1 2 2 2
  spline S142 degree 2 poles (18.5183, 10.1967) (18.5508, 10.371) (18.4738, 10.7335) (18.3667, 10.9176) knots 0 0 0 1 2 2 2
  spline S143 degree 2 poles (18.3667, 10.9176) (18.2642, 11.0937) (17.9665, 11.4028) (17.803, 11.5273) knots 0 0 0 1 2 2 2
  spline S144 degree 2 poles (17.803, 11.5273) (17.6654, 11.6348) (17.3539, 11.8018) (17.2513, 11.8493) knots 0 0 0 1 2 2 2
  line L107 (17.2513, 11.8493) -> (17.2303, 11.8853)
  line L108 (17.2303, 11.8853) -> (17.9348, 12.2952)
  spline S145 degree 2 poles (17.9348, 12.2952) (18.1537, 12.1493) (18.7761, 11.5309) (18.9671, 11.2027) knots 0 0 0 1 2 2 2
  spline S146 degree 2 poles (18.9671, 11.2027) (19.37, 10.5102) (19.0917, 9.3033) (18.4672, 8.94) knots 0 0 0 1 2 2 2
  spline S147 degree 2 poles (18.4672, 8.94) (18.175, 8.7699) (17.6075, 8.6219) (17.3294, 8.6208) knots 0 0 0 1 2 2 2
  spline S148 degree 2 poles (17.3294, 8.6208) (17.0434, 8.6152) (16.4165, 8.7165) (16.1005, 8.7899) knots 0 0 0 1 2 2 2
  spline S149 degree 2 poles (16.1005, 8.7899) (15.5786, 8.9041) (14.4052, 9.2447) (14.0602, 9.3495) knots 0 0 0 1 2 2 2
  line L109 (14.0602, 9.3495) -> (15.4717, 6.9237)
  line L110 (15.4717, 6.9237) -> (14.8993, 6.5906)
  dimension "d112" = 38.1
  constraints: 1 centre point, 1 coincident, 1 other
  measures "d112" diameter of A0
extrude "Extrusion1" cut sketch "Sketch11" against normal blind 1.27
equation "\"d72\" = caseHeightAboveLens"
equation "\"d73\" = a1MajorRadius"
equation "\"d77\" = wallThickness"
equation "\"d78\" = wallThickness"
equation "\"d100\" = threadAngle"
equation "\"d101\" = pitch"
equation "\"d102\" = a1RootRadius"
equation "\"d103\" = a1MinorRadius"
equation "\"d104\" = pitch"
equation "\"baseDiameter\" = 31.75"
equation "\"baseRadius\" = 0.5 * baseDiameter"
equation "\"baseHeight\" = 25.4"
equation "\"middleDiameter\" = 34.29"
equation "\"middleRadius\" = 0.5 * middleDiameter"
equation "\"middleTopDiameter\" = 34.798"
equation "\"middleTopRadius\" = 0.5 * middleTopDiameter"
equation "\"middleHeight\" = 18.542"
equation "\"middleTopHeight\" = 30.734"
equation "\"topBaseDiameter\" = 34.798"
equation "\"topHeightDiameter\" = 40.894"
equation "\"topBaseRadius\" = 0.5 * topBaseDiameter"
equation "\"topHeightRadius\" = 0.5 * topHeightDiameter"
equation "\"topHeight\" = 7.62"
equation "\"d9\" = caseBottomThickness"
equation "\"wallThickness\" = 3.175"
equation "\"caseBottomThickness\" = 4.7625"
equation "\"caseHeightAboveLens\" = 12.7"
equation "\"baseWallThickness\" = 2.032"
equation "\"baseInteriorHeight\" = 15.24"
equation "\"interiorRadius\" = 0.5 * interiorDiameter"
equation "\"outsideRadius\" = interiorRadius + wallThickness"
equation "\"outsideDiameter\" = 2 * outsideRadius"
equation "\"textRingDiameter\" = 0.75 * outsideDiameter"
equation "\"b2MajorDiameterMax\" = 41.275"
equation "\"b2MajorRadiusMax\" = 0.5 * b2MajorDiameterMax"
equation "\"a1MinorDiameter\" = 44.39412"
equation "\"a1MinorRadius\" = 0.5 * a1MinorDiameter"
equation "\"a1MajorDiameter\" = 47.1424"
equation "\"a1MajorRadius\" = 0.5 * a1MajorDiameter"
equation "\"a1RootRadius\" = 0.25908"
equation "\"topThickness\" = 9.525"
equation "\"threadAngle\" = 60deg"
equation "\"pitch\" = 2.116667"
equation "\"interiorDiameter\" = 41.275"
body "Solid3"
